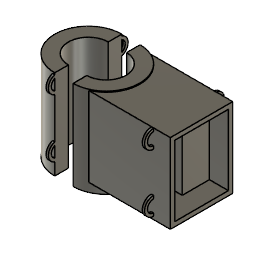
e button holder (Autodesk Fusion 360 design; units mm, degrees)
part number: 2026-04-04-15-37-33-043
Autodesk Fusion 360 part; units mm, degrees
note: some values were not read from the file. Chosen so that the rebuilt part matches the saved one: which face or edge a step refers to; which pieces of a blend or face edit are solid.
sketch "Sketch1" plane through (0, 0, 0) normal (0, 0, 1) x (1, 0, 0)
  circle A0 centre (0, 0) radius 11.303
  circle A1 centre (0, 0) radius 19.05
  dimension "d2" = 22.606
  dimension "d3" = 38.1
  constraint coincident A0.centre A1.centre
  constraint concentric A0 A1
  measures "d2" diameter of A0
  measures "d3" diameter of A1
extrude "Extrude1" add sketch "Sketch1" along normal blind 50.8 makes body 1
sketch "Sketch2" plane through (0, 0, 0) normal (1, 0, 0) x (0, 1, 0)
  line L0 (-14.9987, 47.6936) -> (15.4051, 47.6936)
  line L1 (15.4051, 47.6936) -> (15.4051, 7.6886)
  line L2 (15.4051, 7.6886) -> (-14.9987, 7.6886)
  line L3 (-14.9987, 7.6886) -> (-14.9987, 47.6936)
  line L4 (-14.9987, 47.6936) -> (0, 47.6936)
  line L5 (0, 47.6936) -> (0, 7.6886)
  line L6 (0, 7.6886) -> (-14.9987, 7.6886)
  line L7 (-14.9987, 7.6886) -> (-14.9987, 47.6936)
  line L8 (0, 0) -> (0, 60.211) construction
  line L9 (-17.5387, 50.2336) -> (2.54, 50.2336)
  line L10 (2.54, 50.2336) -> (2.54, 5.08)
  line L11 (2.54, 5.08) -> (-17.5387, 5.08)
  line L12 (-17.5387, 5.08) -> (-17.5387, 50.2336)
  line L13 (-17.5387, 50.2336) -> (17.9451, 50.2336)
  line L14 (17.9451, 50.2336) -> (17.9451, 5.08)
  line L15 (17.9451, 5.08) -> (-17.5387, 5.08)
  line L16 (-17.5387, 5.08) -> (-17.5387, 50.2336)
  circle A0 centre (-17.5387, 29.7109) radius 3.4829
  circle A1 centre (-17.5387, 29.7109) radius 5.1459
  line L17 (-17.4378, 34.8558) -> (-17.4378, 24.566)
  circle A2 centre (-17.5387, 44.9509) radius 3.4829
  circle A3 centre (-17.5387, 44.9509) radius 5.1459
  circle A4 centre (-17.5387, 11.9309) radius 3.4829
  circle A5 centre (-17.5387, 11.9309) radius 5.1459
  circle A6 centre (17.5387, 44.9509) radius 3.4829
  circle A7 centre (17.5387, 44.9509) radius 5.1459
  circle A8 centre (17.5387, 29.7109) radius 3.4829
  circle A9 centre (17.5387, 29.7109) radius 5.1459
  circle A10 centre (17.5387, 11.9309) radius 3.4829
  circle A11 centre (17.5387, 11.9309) radius 5.1459
  point P0 (0, 7.6886)
  dimension "d6" = 30.4038
  dimension "d7" = 40.005
  dimension "d8" = 14.9987
  dimension "d10" = 5.08
  dimension "d11" = 2.54
  dimension "d12" = 2.54
  dimension "d13" = 2.54
  dimension "d14" = 2.54
  dimension "d27" = 6.9659
  dimension "d28" = 10.2918
  dimension "d29" = 6.9659
  dimension "d30" = 10.2918
  dimension "d31" = 6.9659
  dimension "d32" = 10.2918
  constraint horizontal L0
  constraint vertical L1
  constraint horizontal L2
  constraint vertical L3
  constraint horizontal L4
  constraint vertical L5
  constraint horizontal L6
  constraint vertical L7
  constraint coincident L2 P0
  constraint coincident P0 L5.end
  constraint coincident L8.start origin
  constraint perpendicular L2 L8
  constraint coincident P0 L8
  constraint horizontal L9
  constraint vertical L10
  constraint horizontal L11
  constraint vertical L12
  constraint horizontal L13
  constraint vertical L14
  constraint horizontal L15
  constraint vertical L16
  constraint concentric A0 A1
  constraint coincident A1 L17.start
  constraint coincident A1 L17.end
  constraint parallel L10 L17
  constraint coincident L16 A0.centre
  constraint concentric A2 A3
  constraint concentric A4 A5
  constraint symmetric L8 A0 A8
  constraint symmetric L8 A1 A9
  constraint symmetric L8 A2 A6
  constraint symmetric L8 A3 A7
  constraint symmetric L8 A4 A10
  constraint symmetric L8 A5 A11
  measures "d6" distance of L0.start L0.end
  measures "d7" distance of L0.end L1.end
  measures "d8" distance of P0 L2.end
  measures "d10" vertical distance of L8.start L10.end
  measures "d11" distance of L7 L16
  measures "d12" distance of L0 L9
  measures "d13" distance of L8 L10
  measures "d14" distance of L1 L14
  measures "d27" diameter of A0
  measures "d28" diameter of A1
  measures "d29" diameter of A2
  measures "d30" diameter of A3
  measures "d31" diameter of A4
  measures "d32" diameter of A5
extrude "Extrude2" add sketch "Sketch2" along normal blind 35.56 from surface at 7.62 contours L0 L3 L4 L7 L12 L16 A2 A3 | L0 L4 L9 L10 L12 L13 L16 A3 | L3 L7 L12 L16 A2 | L0 L2 L5 L10 | L3 L7 L12 L16 A2 A3 | L2 L6 L10 L11 L12 L15 L16 A5 | L3 L7 L12 L16 A1 A3 | L2 L3 L6 L7 L12 L16 A4 A5 | L3 L7 A0 A1 L17 | L12 L16 A0 A1 L17 | L3 L7 A0 L17 | L12 L16 A0 L17 | L3 L7 L12 L16 A1 A5 | L12 L16 A0 A1 L17 | L3 L7 L12 L16 A4 | L3 L7 L12 L16 A4 A5 | L3 L7 A0 A1 L17 bodies 1
delete_face "DeleteFace1" 1 faces at (7.9798, -4.3415, 50.2336) on bodies 1
extrude "Extrude3" add sketch "Sketch2" along normal blind 35.56 from surface at 7.62 contours L0 L10 L13 L14 A7 | L0 L14 A6 A7 | L2 L10 L14 L15 A11 | L0 L1 L14 A6 | L1 L14 A7 A9 | L1 L14 A6 A7 | L1 L2 L14 A10 A11 | L1 L14 A8 A9 | L1 L14 A10 A11 | L1 L14 A9 A11 | L1 L14 A8 | L1 L14 A8 A9 | L1 L14 A10 bodies 1
extrude "Extrude4" add sketch "Sketch2" along normal blind 5.08 from surface at 38.1 contours L0 L1 L2 L10 A7 A9 A11 | L0 L1 A6 A7 | L0 L1 A6 | L1 L2 A10 A11 | L1 A8 A9 | L1 A8 | L1 A10 bodies 1
extrude "Extrude5" add sketch "Sketch2" along normal blind 10.795 from surface at 43.18 contours L0 L3 L4 L7 L12 L16 A2 A3 | L0 L4 L9 L10 L12 L13 L16 A3 | L3 L7 L12 L16 A2 | L3 L7 L12 L16 A2 A3 | L0 L10 L13 L14 A7 | L2 L6 L10 L11 L12 L15 L16 A5 | L3 L7 L12 L16 A1 A3 | L0 L14 A6 A7 | L2 L10 L14 L15 A11 | L2 L3 L6 L7 L12 L16 A4 A5 | L3 L7 A0 A1 L17 | L12 L16 A0 A1 L17 | L0 L1 L14 A6 | L1 L14 A7 A9 | L1 L14 A6 A7 | L1 L2 L14 A10 A11 | L3 L7 A0 L17 | L12 L16 A0 L17 | L3 L7 L12 L16 A1 A5 | L12 L16 A0 A1 L17 | L1 L14 A8 A9 | L1 L14 A10 A11 | L1 L14 A9 A11 | L3 L7 L12 L16 A4 | L3 L7 L12 L16 A4 A5 | L3 L7 A0 A1 L17 | L1 L14 A8 | L1 L14 A8 A9 | L1 L14 A10 bodies 1
delete_face "DeleteFace2" 1 faces at (9.7537, 2.9765, 50.2336) on bodies 1
delete_face "DeleteFace3" 4 faces at (9.7537, 2.9765, 5.08) (7.62, 4.4761, 5.9495) (8.7513, 2.54, 6.8191) (9.7537, 2.9765, 7.6886) on bodies 1
extrude "Extrude6" add sketch "Sketch2" against normal blind 1.27 contours L12 L16 A0 A1 bodies 1
extrude "Extrude7" add sketch "Sketch2" along normal blind 1.27 from surface at 43.18 contours L12 L16 A2 A3 bodies 1
extrude "Extrude8" add sketch "Sketch2" along normal blind 1.27 from surface at 43.18 contours L12 L16 A4 A5 | L14 A10 A11 bodies 1
extrude "Extrude9" add sketch "Sketch2" along normal blind 1.27 from surface at 43.18 contours L14 A6 A7 bodies 1
extrude "Extrude10" add sketch "Sketch2" against normal blind 1.27 contours L14 A8 A9 bodies 1
delete_face "DeleteFace4" 1 faces at (0, -19.7502, 25.7007) on bodies 1
delete_face "DeleteFace5" 1 faces at (-0.4233, 22.6846, 29.7109) on bodies 1
extrude "Extrude11" add sketch "Sketch2" against normal blind 1.27 contours L12 L16 A2 A3 | L14 A6 A7 | L12 L16 A4 A5 | L14 A10 A11 bodies 1
sketch "Sketch3" plane through (0, 0, 0) normal (1, 0, 0) x (0, 1, 0)
  line L0 (-26.0283, 54.6918) -> (25.5981, 54.6918)
  line L1 (25.5981, 54.6918) -> (25.5981, -5.1089)
  line L2 (25.5981, -5.1089) -> (-26.0283, -5.1089)
  line L3 (-26.0283, -5.1089) -> (-26.0283, 54.6918)
  constraint horizontal L0
  constraint vertical L1
  constraint horizontal L2
  constraint vertical L3
extrude "Extrude12" cut sketch "Sketch3" along normal blind 0.254 bodies 1 makes body 2 at (-4.189, 18.5837, 22.5542)
move_body "Move1" bodies 2 to x (1, 0, 0) y (0, 1, 0) z (0, 0, 1) at (-10.16, 0, 0)
